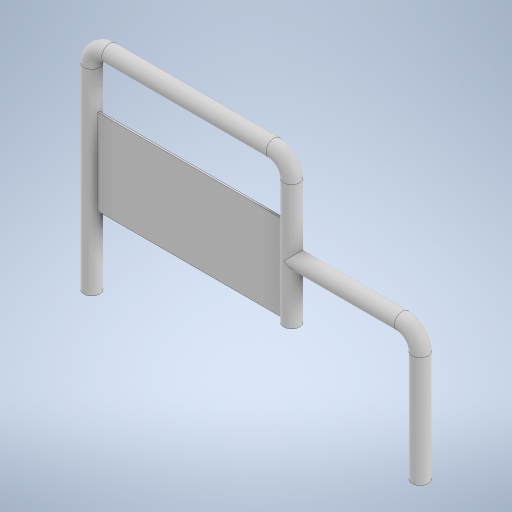
# Autodesk Inventor part: frame of armrest
Saved by Autodesk Inventor 2023 (Build 270158000, 158)
## iProperties
Created: 2023-10-18
Part Number: frame of armrest
Material: Generic
Document SubType Name: Modeling
Designer: tbc
Density: 1 g/cm^3
Appearance: Default
Author: tbc
Autodesk Inventor part; units mm, degrees
ref_plane "YZ Plane" through (0, 0, 0) normal (1, 0, 0) x (0, 1, 0)
ref_plane "XY Plane" through (0, 0, 0) normal (0, 0, 1) x (1, 0, 0)
sketch "Sketch1" plane through (0, 0, 0) normal (0, 0, 1) x (1, 0, 0)
  line L0 (0, 0) -> (0, 275)
  line L1 (25, 300) -> (255, 300)
  line L2 (280, 275) -> (280, 180)
  line L3 (280, 180) -> (435, 180)
  line L4 (460, 155) -> (460, 0)
  arc A0 (25, 300) -> (0, 275) centre (25, 275) ccw
  arc A1 (280, 275) -> (255, 300) centre (255, 275) ccw
  arc A2 (460, 155) -> (435, 180) centre (435, 155) ccw
  line L5 (280, 180) -> (280, 93.2639)
  point P0 (0, 300)
  point P1 (280, 300)
  point P2 (460, 180)
  dimension "d0" = 300
  dimension "d1" = 280
  dimension "d2" = 120
  dimension "d3" = 180
  dimension "d4" = 25
  dimension "d5" = 25
  dimension "d6" = 25
  dimension "d7" = 86.7361
  constraints: 12 end point, 6 point on circle, 6 point on line, 6 tangent, 4 vertical, 3 centre point, 2 horizontal
  measures "d0" distance of L0.start point (0, 300)
  measures "d1" distance of point (0, 300) point (280, 300)
  measures "d2" distance of point (280, 300) L2.end
  measures "d3" distance of L2.end point (460, 180)
  measures "d4" radius of A0
  measures "d5" radius of A1
  measures "d6" radius of A2
  measures "d7" distance of L2.end L5.end
sketch "Sketch2" plane through (0, 0, 0) normal (0, 1, 0) x (-1, 0, 0)
  circle A0 centre (0, 0) radius 11.25
  dimension "d8" = 22.5
  constraints: 1 centre point, 1 coincident
  measures "d8" diameter of A0
sweep "Sweep1" add profiles "Sketch2" path "Sketch1" path curves L0 A0 L1 A1 L2 L3 A2 L4
sketch "Sketch3" plane through (0, 0, 0) normal (0, 1, 0) x (-1, 0, 0)
  point P0 (0, 0)
sketch "Sketch4" plane through (0, 0, 0) normal (0, 0, 1) x (1, 0, 0)
  line L0 (280, 180) -> (280, 180) projected
  line L1 (280, 180) -> (280, 100)
  point P0 (0, 0)
  dimension "d11" = 80
  constraints: 2 end point, 1 vertical
  measures "d11" distance of L0.start L1.end
ref_plane "Work Plane1" through (0, 100, 0) normal (0, 1, 0) x (-1, 0, 0)
sketch "Sketch5" plane through (0, 100, 0) normal (0, 1, 0) x (-1, 0, 0)
  circle A0 centre (-280, 0) radius 11.25 projected
  circle A1 centre (-280, 0) radius 11.25
  point P0 (0, 0)
  dimension "d13" = 22.5
  constraints: 1 centre point, 1 coincident
  measures "d13" diameter of A1
sweep "Sweep2" add profiles "Sketch5" path "Sketch4" path curves L1
sketch "Sketch6" plane through (0, 0, 0) normal (0, 0, 1) x (1, 0, 0)
  line L0 (0, 101.8033) -> (281.8033, 101.8033)
  line L1 (281.8033, 101.8033) -> (281.8033, 221.8033)
  line L2 (281.8033, 221.8033) -> (0, 221.8033)
  line L3 (0, 221.8033) -> (0, 101.8033)
  point P0 (0, 0)
  dimension "d16" = 120
  constraints: 8 end point, 2 parallel, 1 horizontal, 1 perpendicular
  measures "d16" distance of L2.end L0.start
extrude "Extrusion1" add sketch "Sketch6" along normal blind 2.5
body "Solid1"
